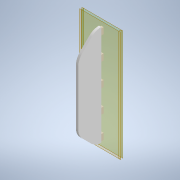
# Autodesk Inventor part: middle
Saved by Autodesk Inventor 2020 (Build 240168000, 168)
## iProperties
Created: 2020-03-09
Part Number: middle
Material: Generic
Document SubType Name: Modeling
Designer: erwin
Density: 1 g/cm^3
Appearance: Default
Author: erwin
Autodesk Inventor part; units mm, degrees
ref_plane "YZ Plane" through (0, 0, 0) normal (1, 0, 0) x (0, 1, 0)
ref_plane "XZ Plane" through (0, 0, 0) normal (0, 1, 0) x (-1, 0, 0)
ref_plane "XY Plane" through (0, 0, 0) normal (0, 0, 1) x (1, 0, 0)
ref_plane "Work Plane3" through (0, -195, 0) normal (-1, 0, 0) x (0, 0, 1)
ref_plane "Work Plane1" through (72.5, 195, 0) normal (1, 0, 0) x (0, 0, -1)
ref_plane "Work Plane2" through (-72.5, -195, 0) normal (-1, 0, 0) x (0, 0, 1)
ref_plane "Work Plane4" through (0, 0, 0) normal (0, 0, 1) x (1, 0, 0)
sketch "Sketch1" plane through (0, -195, 0) normal (-1, 0, 0) x (0, 0, 1)
  line L0 (0, 0) -> (0, 390) projected
  line L1 (0, 390) -> (-9, 390) projected
  line L2 (-9, 0) -> (-9, 390) projected
  line L3 (0, 0) -> (-9, 0) projected
  arc A0 (0, 0) -> (38.6396, 16.0051) centre (0, 54.6447) ccw
  line L4 (38.6396, 16.0051) -> (73.9949, 51.3604)
  arc A1 (73.9949, 51.3604) -> (90, 90) centre (35.3553, 90) ccw
  line L5 (90, 90) -> (90, 195)
  line L6 (0, 0) -> (0, 195)
  line L7 (90, 195) -> (-62.3705, 195) construction
  line L8 (0, 390) -> (-9, 390)
  arc A2 (38.6396, 373.9949) -> (0, 390) centre (0, 335.3553) ccw
  line L9 (38.6396, 373.9949) -> (73.9949, 338.6396)
  arc A3 (90, 300) -> (73.9949, 338.6396) centre (35.3553, 300) ccw
  line L10 (90, 300) -> (90, 195)
  line L11 (0, 390) -> (0, 195)
  dimension "d0" = 90
  dimension "d1" = 45
  dimension "d2" = 50
  constraints: 16 end point, 8 point on circle, 5 symmetric about line, 4 centre point, 4 tangent, 1 collinear, 1 equal radius, 1 horizontal, 1 vertical, 2 other
  measures "d0" distance between parallel lines of L0 L5
  measures "d1" angle of L0 L4
  measures "d2" distance of L4.start L4.end
extrude "Extrusion1" add sketch "Sketch1" along normal mid plane 9 contours L0 A2 L9 A3 L10 L5 A1 L4 A0
ref_plane "Work Plane5" through (0, 0, -9) normal (0, 0, -1) x (-1, 0, 0)
sketch "Sketch2" plane through (0, 0, -9) normal (0, 0, -1) x (-1, 0, 0)
  line L0 (-4.5, -195) -> (4.5, -195) projected
  line L1 (4.5, 195) -> (4.5, -195) projected
  line L2 (-4.5, 195) -> (4.5, 195) projected
  line L3 (-4.5, -195) -> (-4.5, 195) projected
  line L4 (4.5, 195) -> (4.5, -195) projected
  line L5 (-4.5, -195) -> (-4.5, 195) projected
  line L6 (4.5, -180) -> (-4.5, -180)
  line L7 (-4.5, -180) -> (-4.5, -156)
  line L8 (-4.5, -156) -> (4.5, -156)
  line L9 (4.5, -156) -> (4.5, -180)
  line L10 (4.5, -105) -> (4.5, 105) projected
  line L11 (-4.5, 105) -> (-4.5, -105) projected
  line L12 (4.5, -96) -> (-4.5, -96)
  line L13 (-4.5, -96) -> (-4.5, -72)
  line L14 (-4.5, -72) -> (4.5, -72)
  line L15 (4.5, -72) -> (4.5, -96)
  point P0 (0, 0)
  point P1 (4.5, -156)
  point P2 (-4.5, -156)
  point P3 (-4.5, -180)
  point P4 (-4.5, -96)
  point P5 (4.5, -96)
  dimension "d5" = 24
  dimension "d6" = 24
  dimension "d7" = 15
  dimension "d8" = 60
  constraints: 16 end point, 4 parallel, 4 point on line, 2 horizontal, 2 perpendicular
  measures "d5" distance of L6.end L7.end
  measures "d6" distance of L12.end L13.end
  measures "d7" distance from line of L0.end L6
  measures "d8" distance between parallel lines of L12 L8
extrude "Extrusion2" add sketch "Sketch2" against normal blind 9 contours L3 L8 L1 L6 | L3 L14 L1 L12
mirror "Mirror1" about plane through (0, 0, 0) normal (0, 1, 0) of "Extrusion2"
sketch "Sketch3" plane through (4.5, -72, 0) normal (0, 0, -1) x (-1, 0, 0)
  line L0 (9, 144) -> (9, 0) projected
  line L1 (0, 84) -> (9, 84)
  line L2 (9, 84) -> (9, 60)
  line L3 (9, 60) -> (0, 60)
  line L4 (0, 60) -> (0, 84)
  line L5 (0, 84) -> (9, 60) construction
  line L6 (9, 84) -> (0, 60) construction
  point P0 (4.5, 72)
  dimension "d11" = 24
  constraints: 12 end point, 2 midpoint, 2 parallel, 1 horizontal, 1 perpendicular, 1 point on line
  measures "d11" distance of L1.end L2.end
extrude "Extrusion3" add sketch "Sketch3" along normal blind 9
sketch "Sketch4" plane through (-4.5, -195, 0) normal (-1, 0, 0) x (0, 0, 1)
  point P0 (0, 195)
body "Solid1"
